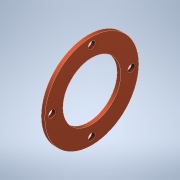
# Autodesk Inventor part: flatza
Saved by Autodesk Inventor 2021 (Build 250183000, 183)
## iProperties
Created: 2020-12-28
Part Number: flatza
Material: Copper
Document SubType Name: Sheet Metal
Designer: Διογενης Τσιχλακης
Density: 8.94 g/cm^3
Sheet Metal Rule: Default_mm
Appearance: Copper - Satin
Author: Διογενης Τσιχλακης
Autodesk Inventor part; units mm, degrees
ref_plane "YZ Plane" through (0, 0, 0) normal (1, 0, 0) x (0, 1, 0)
ref_plane "XZ Plane" through (0, 0, 0) normal (0, 1, 0) x (-1, 0, 0)
ref_plane "XY Plane" through (0, 0, 0) normal (0, 0, 1) x (1, 0, 0)
sketch "Sketch1" plane through (0, 0, 0) normal (1, 0, 0) x (0, 1, 0)
  circle A0 centre (55, 0) radius 5
  circle A1 centre (0, 0) radius 40
  circle A2 centre (0, 0) radius 65
  circle A3 centre (0, 55) radius 5
  circle A4 centre (-55, 0) radius 5
  circle A5 centre (0, -55) radius 5
  dimension "d1" = 10
  dimension "d2" = 80
  dimension "d3" = 130
  dimension "d8" = 360
  constraints: 6 centre point, 1 coincident, 9 other
  measures "d1" diameter of A0
  measures "d2" diameter of A1
  measures "d3" diameter of A2
extrude "Extrusion1" add sketch "Sketch1" against normal blind 5
equation "\"BendRadius\" = Thickness"
equation "\"BendReliefWidth\" = Thickness"
equation "\"BendReliefDepth\" = 0.5 * Thickness"
equation "\"CornerReliefSize\" = 4 * Thickness"
equation "\"MinimumRemnant\" = 2 * Thickness"
equation "\"TransitionRadius\" = BendRadius"
equation "\"JacobiRadiusSize\" = BendRadius"
equation "\"GapSize\" = Thickness"
equation "\"Thickness\" = 0.5"
body "Solid1"
